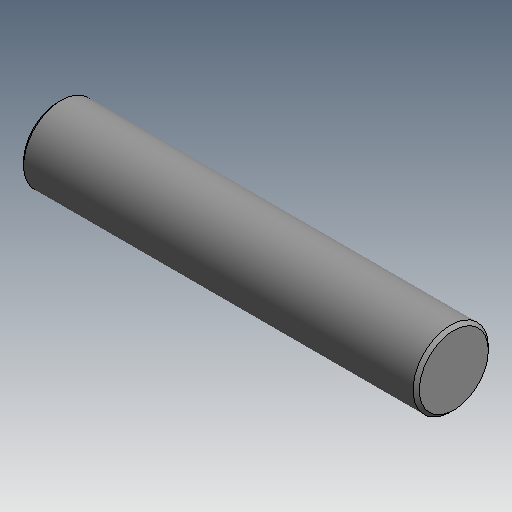
# Autodesk Inventor part: PSSFG12-63-RC22
Saved by Autodesk Inventor 2020 (Build 240168000, 168)
## iProperties
Part Number: PSSFG12-63-RC22
Material: 一般
Catalog Web Link: www.cadenas.de
Description: SFJ, SFU, SSFJ, SSFU, PSFJ, PSFU, PSSFJ, PSSFU, RSFJ, PSFG, PSSFG-Shafts - Solid Type
Vendor: MISUMI
Document SubType Name: Modeling
Designer: partserver
Manufacturer: MISUMI
Mass: 7.06195 g
Surface Area: 25.9177 cm^2
Volume: 7.06195 cm^3
Density: 1 g/cm^3
Appearance: PSOLRGB-175-175-175
Category: PARTsolutions
Company: MISUMI
PSOL_IDENT_0: {$CADENAS_DATA\23d-libs\misumi\metric\01_linear_shafts\sfj.prj},378 {VTYP=3D},{NB=PSSFG12-63-RC22},{
PSOL_IDENT_1: LINA=PSSFG12-63-RC22},{NN=SFJ, SFU, SSFJ, SSFU, PSFJ, PSFU, PSSFJ, PSSFU, RSFJ, PSFG, PSSFG},{DATE=0
PSOL_IDENT_2: 6.07.2021 09:52:54},{GEOMDATE=14.05.2021 06:14:48},{VERSION=},{LINEID=70},{WBVAR=DTS,MAT,ST,ALT1,L,A
PSOL_IDENT_3: LT3,SC,WSC,X,ALT4,FC,WFC,A,E,ALT5,RC,WRC,Y,ALT6,VC,WVC,F,ALT7,KC,G,WKC,CALT7},{WBNUMERIC=L,SC,WSC,X,
PSOL_IDENT_4: FC,WFC,A,E,RC,WRC,Y,VC,WVC,F,KC,G,WKC,CALT7}  {NB=PSSFG12-63-RC22},{LINA=PSSFG12-63-RC22},{KT=DUMMY}
PSOL_IDENT_5: ,{PN=PSSFG12-63-RC22},{TYPE=PSSFG},{DTS=f8},{DTSALG= 'g6','g6' , 'h5','h5' , 'f8','f8' },{MAT=SUS304
PSOL_IDENT_6: },{MATALG= 'S45C','S45C Equivalent','SUS304','304 Stainless Steel' },{ST=HCP10},{STALG= 'HCP10','Har
PSOL_IDENT_7: d Chrome Plating Plating Hardness: HV750 ~ Plating Thickness: 10 microns or More' },{D=12},{ALT1=},{
PSOL_IDENT_8: ALT1ALG= '','w/o LKC (L Dimension Tolerance Change)','LKC','with LKC (L Dimension Tolerance Change)'
PSOL_IDENT_9: },{ALT1PN=},{L=63.0},{LALG=[15:1400/1]},{LMIN=15},{LMAX=1400},{C=0.5},{ALT3=},{ALT3ALG= '','w/o Wre
PSOL_IDENT_10: nch Flats' , 'SC','with SC (Wrench Flats at One Location)' , 'WSC','with WSC (Wrench Flats at Two Lo
PSOL_IDENT_11: cations)' },{ALT3PN=},{SC=0},{SCALG=[0]},{SCMAX=53},{WSC=0},{WSCALG=[0]},{WSCMAX=41},{X=0},{XALG=[0]
PSOL_IDENT_12: },{XMAX=41},{WALT3=0},{LL1=0},{LL1ALG=10},{ALT4=},{ALT4ALG= '','w/o Set Screw Flat','FC','with FC (S
PSOL_IDENT_13: et Screw Flat at One Location)','WFC','with WFC (Set Screw Flats at Two Locations)' },{ALT4PN=},{FC=
PSOL_IDENT_14: 0},{FCALG=[0]},{FCMAX=60},{WFC=0},{WFCALG=[0]},{WFCMAX=30},{A=0},{AALG=[0]},{AMAX=0},{E=0},{EALG=[0]
PSOL_IDENT_15: },{EMAX=61},{HHALT4=0.0},{CIFA=0},{CIFE=0},{FC3D=0},{ALT5=RC},{ALT5ALG= '','w/o 90-deg. Set Screw Fl
PSOL_IDENT_16: at','RC','with RC (90-deg. Set Screw Flat at One Location)','WRC','with WRC (90-deg. Set Screw Flats
PSOL_IDENT_17: at Two Locations)' },{ALT5PN=-RC22},{RC=22},{RCALG=[2:57/1]},{RCMIN=2},{RCMAX=57},{WRC=0},{WRCALG=[
PSOL_IDENT_18: 0]},{WRCMIN=2},{WRCMAX=47},{Y=0},{YALG=[0]},{YMIN=2},{YMAX=49},{BB1=6},{BB1ALG=6},{HHALT5=1.0},{ALT6=
PSOL_IDENT_19: },{ALT6ALG= '','w/o V Groove','VC','with VC (V Groove at One Location)','WVC','with WVC (V Grooves a
PSOL_IDENT_20: t Two Locations)' },{ALT6PN=},{VC=0},{VCALG=[0]},{VCMIN=5},{VCMAX=61},{WVC=0},{WVCALG=[0]},{WVCMIN=2
PSOL_IDENT_21: },{WVCMAX=56},{F=0},{FALG=[0]},{FMIN=5},{FMAX=61},{WALT6=0},{WALT6ALG=4},{ALT7=},{ALT7ALG= '','w/o A
PSOL_IDENT_22: dd keyway','KC','with KC (Add keyway at one location)','WKC','with WKC (Adds Keyways at two location
PSOL_IDENT_23: s)' },{ALT7PN=},{KC=0},{KCALG=[0]},{KCMAX1=61},{KCMAX2=63},{KCMAX3=61},{G=0},{GALG=[0]},{GMIN=0},{GM
PSOL_IDENT_24: AX1=60},{GMAX2=60},{GMAX3=60},{WKC=0},{WKCALG=[0]},{WKCMAX=61},{CALT7=0},{CALT7ALG=[0]},{CALT7MIN=0}
PSOL_IDENT_25: ,{CALT7MAX=60},{BB=0},{TT=0.0},{CIFKC=0},{CIFWKC=0},{ERRORPN=},{ERRORALT34=OK},{ERRORALT35=OK},{ERRO
PSOL_IDENT_26: RALT36=OK},{ERRORALT37=OK},{ERRORALT45=OK},{ERRORALT46=OK},{ERRORALT47=OK},{ERRORALT56=OK},{ERRORALT
PSOL_IDENT_27: 57=OK},{ERRORALT67=OK},{FONTSIZE=1.080}
NB: PSSFG12-63-RC22
NN: SFJ, SFU, SSFJ, SSFU, PSFJ, PSFU, PSSFJ, PSSFU, RSFJ, PSFG, PSSFG
NT: Shafts - Solid Type
NBSYN: $PN.
LINA: PSSFG12-63-RC22
CATALOG: Misumi
PN: PSSFG12-63-RC22
DTS: f8
MAT: 304 Stainless Steel
ST: Hard Chrome Plating Plating Hardness: HV750 ~ Plating Thickness: 10 microns or More
D: 12
ALT1: w/o LKC (L Dimension Tolerance Change)
L: 63
C: 0.5
ALT3: w/o Wrench Flats
SC: 0
WSC: 0
X: 0
WALT3: 0
LL1: 0
ALT4: w/o Set Screw Flat
FC: 0
WFC: 0
A: 0
E: 0
HHALT4: 0
ALT5: with RC (90-deg. Set Screw Flat at One Location)
RC: 22
WRC: 0
Y: 0
BB1: 6
HHALT5: 1
ALT6: w/o V Groove
VC: 0
WVC: 0
F: 0
WALT6: 0
ALT7: w/o Add keyway
KC: 0
G: 0
WKC: 0
CALT7: 0
BB: 0
TT: 0
SUPPLIER: MISUMI
ARTICLENO: PSSFG12-63-RC22
BOMINFO: PSSFG12-63-RC22
CREATOR: CADENAS GmbH
Title: PSSFG12-63-RC22
Author: Cadenas PARTsolutions
Comments: Shafts - Solid Type
Autodesk Inventor part; units mm, degrees
ref_plane "YZ Plane" through (0, 0, 0) normal (1, 0, 0) x (0, 1, 0)
ref_plane "XZ Plane" through (0, 0, 0) normal (0, 1, 0) x (-1, 0, 0)
ref_plane "XY Plane" through (0, 0, 0) normal (0, 0, 1) x (1, 0, 0)
sketch "Sketch_3" plane through (0, 0, 0) normal (0, 0, 1) x (1, 0, 0)
  line L0 (63, 0) -> (0, 0)
  line L1 (0, 0) -> (0, 5.5)
  line L2 (0, 5.5) -> (0.5, 6)
  line L3 (0.5, 6) -> (62.5, 6)
  line L4 (62.5, 6) -> (63, 5.5)
  line L5 (63, 5.5) -> (63, 0)
  line L6 (63, 0) -> (0, 0)
  constraints: 14 end point
revolve "Revolution1" add sketch "Sketch_3" angle 360 about axis through (63, 0, 0) along (1, 0, 0)
sketch "Sketch_10" plane through (22, 0, 0) normal (1, 0, 0) x (0, 0, -1)
  line L0 (-12, 12) -> (-12, -12)
  line L1 (-12, -12) -> (-5, -12)
  line L2 (-5, -12) -> (-5, 5)
  line L3 (-5, 5) -> (12, 5)
  line L4 (12, 5) -> (12, 12)
  line L5 (12, 12) -> (-12, 12)
  constraints: 12 end point
extrude "Extrusion1" cut sketch "Sketch_10" along normal blind 6
body "Solid1"
